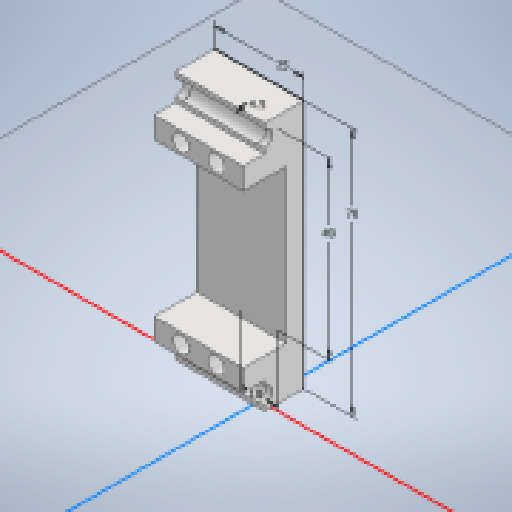
# Autodesk Inventor part: Servo_mount_front
Saved by Autodesk Inventor 2025.2 (Build 292293000, 293)
## iProperties
Created: 2025-01-12
Part Number: Servo_mount_front
Material: Generic
Document SubType Name: Modeling
Designer: caomi
Density: 1 g/cm^3
Appearance: Default
Author: caomi
Autodesk Inventor part; units mm, degrees
ref_plane "YZ Plane" through (0, 0, 0) normal (1, 0, 0) x (0, 1, 0)
ref_plane "XZ Plane" through (0, 0, 0) normal (0, 1, 0) x (-1, 0, 0)
ref_plane "XY Plane" through (0, 0, 0) normal (0, 0, 1) x (1, 0, 0)
sketch "Sketch1" plane through (0, 0, 0) normal (0, 0, 1) x (1, 0, 0)
  line L0 (12.5, -35) -> (-12.5, -35)
  line L1 (-12.5, -35) -> (-12.5, 35)
  line L2 (-12.5, 35) -> (12.5, 35)
  line L3 (12.5, 35) -> (12.5, -35)
  line L4 (12.5, -35) -> (-12.5, 35) construction
  line L5 (-12.5, -35) -> (12.5, 35) construction
  line L6 (5, -24.5) -> (-5, -24.5) construction
  line L7 (-5, -24.5) -> (-5, 24.5) construction
  line L8 (-5, 24.5) -> (5, 24.5) construction
  line L9 (5, 24.5) -> (5, -24.5) construction
  line L10 (5, -24.5) -> (-5, 24.5) construction
  line L11 (-5, -24.5) -> (5, 24.5) construction
  circle A0 centre (-5, 24.5) radius 2.25
  circle A1 centre (5, 24.5) radius 2.25
  circle A2 centre (5, -24.5) radius 2.25
  circle A3 centre (-5, -24.5) radius 2.25
  point P0 (0, 0)
  dimension "d0" = 4.5
  dimension "d1" = 10
  dimension "d2" = 49
  dimension "d3" = 25
  dimension "d4" = 70
  constraints: 24 end point, 4 centre point, 4 coincident, 4 midpoint, 4 parallel, 3 equal radius, 2 horizontal, 2 perpendicular
  measures "d0" diameter of A0
  measures "d1" distance of L6.start L6.end
  measures "d2" distance of L8.end L6.start
  measures "d3" distance of L1.end L2.end
  measures "d4" distance of L2.end L0.start
extrude "Extrusion1" add sketch "Sketch1" along normal blind 5
sketch "Sketch2" plane through (12.5, -35, 0) normal (1, 0, 0) x (0, 0, -1)
  line L0 (-5, 70) -> (-11, 70)
  line L1 (-11, 70) -> (-11, 62.5)
  line L2 (-11, 62.5) -> (-5, 62.5)
  line L3 (-5, 62.5) -> (-5, 70)
  circle A0 centre (-11, 66.25) radius 2.5
  line L4 (2.8141, 35) -> (-33.1304, 35) construction
  line L5 (0, 0) -> (0, 70) projected
  line L6 (-5, 0) -> (-11, 0)
  line L7 (-11, 0) -> (-11, 7.5)
  line L8 (-11, 7.5) -> (-5, 7.5)
  line L9 (-5, 7.5) -> (-5, 0)
  circle A1 centre (-11, 3.75) radius 2.5
  line L10 (-5, 62.5) -> (-17, 62.5)
  line L11 (-17, 62.5) -> (-17, 56.5)
  line L12 (-17, 56.5) -> (-5, 56.5)
  line L13 (-5, 56.5) -> (-5, 62.5)
  line L14 (-5, 7.5) -> (-17, 7.5)
  line L15 (-17, 7.5) -> (-17, 13.5)
  line L16 (-17, 13.5) -> (-5, 13.5)
  line L17 (-5, 13.5) -> (-5, 7.5)
  circle A2 centre (-11, 66.25) radius 2.3
  circle A3 centre (-11, 3.75) radius 2.3
  point P0 (0, 35)
  point P1 (0, 35)
  point P2 (-11, 68.75)
  point P3 (-11, 63.75)
  point P4 (-11, 6.25)
  point P5 (-11, 1.25)
  point P6 (-11, 6.05)
  point P7 (-11, 1.45)
  point P8 (-11, 68.55)
  point P9 (-11, 63.95)
  dimension "d7" = 6
  dimension "d8" = 7.5
  dimension "d9" = 5
  dimension "d12" = 6
  dimension "d13" = 12
  dimension "d16" = 0.2
  constraints: 34 end point, 8 symmetric about line, 4 centre point, 4 parallel, 3 horizontal, 2 midpoint, 2 perpendicular, 1 point on line, 2 other
  measures "d7" distance of L0.start L0.end
  measures "d8" distance of L0.end L1.end
  measures "d9" diameter of A0
  measures "d12" distance of L10.end L11.end
  measures "d13" distance of L2.end L10.end
  measures "d16" radial gap between concentric circles of A2 A0
extrude "Extrusion2" add sketch "Sketch2" against normal up to surface (25 mm away) contours L3 L2 L1 A0 L0 | L13 L12 L11 L10 L2 | L6 L7 A1 L8 L9 | L8 L14 L15 L16 L17
extrude "Extrusion3" cut sketch "Sketch1" along normal up to surface (17 mm away) contours A0 | A1 | A2 | A3
extrude "Extrusion4" add sketch "Sketch2" against normal blind 2 contours A0 L1 A2 | L7 A3 A1 picked at (-9.3509, 68.0205) picked at (-8.6068, 3.394)
mirror "Mirror1" about plane through (0, 0, 0) normal (1, 0, 0) of "Extrusion4"
sketch "Sketch3" plane through (0, 0, 0) normal (0, 0, -1) x (-1, 0, 0)
  circle A0 centre (-5, 24.5) radius 2.75
  circle A1 centre (-5, 24.5) radius 2.25 projected
  line L0 (-5, 24.5) -> (-5, 16.1694) construction
  line L1 (-5, 24.5) -> (-0.8082, 24.5) construction
  circle A2 centre (-5, -24.5) radius 2.75
  circle A3 centre (5, 24.5) radius 2.75
  circle A4 centre (5, -24.5) radius 2.75
  circle A5 centre (5, 24.5) radius 2.25 projected
  circle A6 centre (5, -24.5) radius 2.25 projected
  circle A7 centre (-5, -24.5) radius 2.25 projected
  point P0 (0, 0)
  dimension "d19" = 5.5
  dimension "d22" = 49
  dimension "d25" = 10
  constraints: 4 centre point, 4 end point, 2 horizontal, 2 vertical, 1 concentric, 6 other
  measures "d19" diameter of A0
  measures "d22" distance of A0.centre A2.centre
  measures "d25" distance of A0.centre A3.centre
extrude "Extrusion5" cut sketch "Sketch3" against normal blind 2.8
equation "\"d13\" = 2 * d7"
equation "\"d14\" = d2"
body "Solid1"
